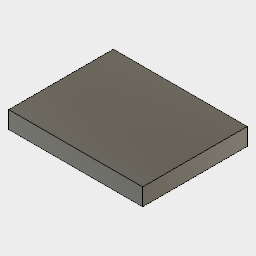
328 2500mAh battery (Autodesk Fusion 360 design; units mm, degrees)
Autodesk Fusion 360 part; units mm, degrees
sketch "Sketch1" plane through (0, 0, 0) normal (0, 0, 1) x (1, 0, 0)
  line L0 (0, 0) -> (61, 0)
  line L1 (61, 0) -> (61, -47.7)
  line L2 (61, -47.7) -> (0, -47.7)
  line L3 (0, -47.7) -> (0, 0)
  dimension "d1" = 61
  dimension "d2" = 47.7
  measures "d1" distance of L0.start L0.end
  measures "d2" distance of L0.start L2.end
extrude "Extrude1" add sketch "Sketch1" along normal blind 7.9
